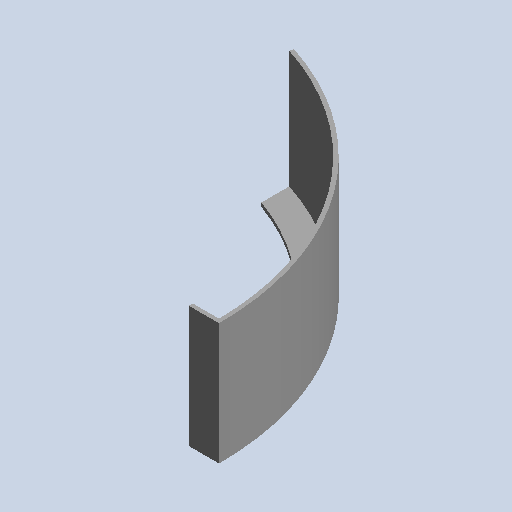
# Autodesk Inventor part: Bottom_Enclosure_1
Saved by Autodesk Inventor 2026 (Build 300175050, 175E)
## iProperties
Part Number: Bottom_Enclosure_1
Material: Generic
Document SubType Name: Modeling
Designer: Kartik
Mass: 96.9988 g
Surface Area: 668.972 cm^2
Volume: 96.9988 cm^3
Density: 1 g/cm^3
Appearance: Default
Author: Kartik
Autodesk Inventor part; units mm, degrees
ref_plane "YZ Plane" through (0, 0, 0) normal (1, 0, 0) x (0, 1, 0)
ref_plane "XZ Plane" through (0, 0, 0) normal (0, 1, 0) x (-1, 0, 0)
ref_plane "XY Plane" through (0, 0, 0) normal (0, 0, 1) x (1, 0, 0)
sketch "Sketch1" plane through (0, 0, 0) normal (0, 1, 0) x (-1, 0, 0)
  arc A0 (-220, 0) -> (-67, -209.5495) centre (0, 0) ccw
  arc A1 (-217, 0) -> (-67, -206.3977) centre (0, 0) ccw
  line L0 (-220, 0) -> (-217, 0)
  line L1 (0, -220) -> (0, -217)
  line L2 (0, -220) -> (-67, -220)
  line L3 (0, -220) -> (67, -220) construction
  line L4 (-67, -220) -> (-67, -206.3977)
  line L5 (-67, -206.3977) -> (-65.0308, -207.0265)
  line L6 (-67, -206.3977) -> (-68.4601, -210.9695)
  point P0 (-67.9127, -209.2555)
  dimension "d0" = 440
  dimension "d1" = 3
  dimension "d2" = 67
  dimension "d3" = 180
  dimension "d9" = 90
  constraints: 14 end point, 4 point on circle, 3 horizontal, 2 centre point, 2 perpendicular, 1 coincident, 1 collinear, 1 point on line
  measures "d0" diameter of A0
  measures "d1" radial gap between concentric circles of A0 A1
  measures "d2" distance of L1.start L2.end
  measures "d3" angle of L2 L3
  measures "d9" angle of L5 L6
extrude "Extrusion1" add sketch "Sketch1" along normal blind 92.5 contours L0 A1 L6 A0
sketch "Sketch2" plane through (0, 0, 0) normal (0, -1, 0) x (1, 0, 0)
  arc A0 (67, -206.3977) -> (217, 0) centre (0, 0) ccw projected
  arc A1 (60.8249, -187.3748) -> (197, 0) centre (0, 0) ccw
  line L0 (197, 0) -> (217, 0)
  line L1 (60.8249, -187.3748) -> (67, -206.3977)
  dimension "d6" = 20
  constraints: 4 end point, 2 point on circle, 1 centre point, 1 horizontal
  measures "d6" radial gap between concentric circles of A0 A1
extrude "Extrusion2" add sketch "Sketch2" against normal blind 3
sketch "Sketch7" plane through (0, 0, 0) normal (0, -1, 0) x (1, 0, 0)
  arc A0 (60.8249, -187.3748) -> (197, 0) centre (0, 0) ccw projected
  arc A1 (67.9127, -209.2555) -> (220, 0) centre (0, 0) ccw projected
  line L0 (197, 0) -> (220, 0) projected
  line L1 (196.9772, -3) -> (219.9795, -3)
  dimension "d28" = 3
  constraints: 2 end point, 2 point on circle, 1 horizontal
  measures "d28" distance between parallel lines of L0 L1
extrude "Extrusion6" add sketch "Sketch7" against normal up to surface (92.5 mm away)
sketch "Sketch8" plane through (0, 3, 0) normal (0, 1, 0) x (1, 0, 0)
  arc A0 (196.9772, 3) -> (60.8249, 187.3748) centre (0, 0) ccw projected
  line L0 (67, 206.3977) -> (60.8249, 187.3748) projected
  line L1 (67, 206.3977) -> (67, 185.2566)
  line L2 (67, 206.3977) -> (88.1411, 206.3977) construction
  dimension "d31" = 90
  constraints: 4 end point, 1 horizontal, 1 perpendicular, 1 point on circle
  measures "d31" angle of L1 L2
extrude "Extrusion7" cut sketch "Sketch8" against normal blind 10
body "Solid1"
